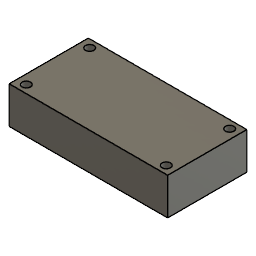
control_dcdc_v0_1 (Autodesk Fusion 360 design; units mm, degrees)
part number: 2026-05-28-15-22-03-641
Autodesk Fusion 360 part; units mm, degrees
box "长方体基本要素1" add length 30 width 60 height 14 placed x (0, 0, 1) y (1, 0, 0) z (0, 1, 0) at (0, 0, 0)
sketch "草图2" plane through (0, 14, 0) normal (0, 1, 0) x (-1, 0, 0)
  line L0 (0, 30) -> (-60, 30)
  line L1 (-60, 30) -> (-60, 0)
  line L2 (-60, 0) -> (0, 0)
  line L3 (0, 0) -> (0, 30)
  circle A0 centre (-3.5, 3) radius 1.6
  circle A1 centre (-3.5, 27) radius 1.6
  circle A2 centre (-56.5, 3) radius 1.6
  circle A3 centre (-56.5, 27) radius 1.6
  line L4 (3.6215, 15) -> (-73.595, 15) construction
  line L5 (-30, -5.3507) -> (-30, 35.2179) construction
  point P0 (0, 15)
  point P1 (-30, 0)
  dimension "d8" = 3.2
  dimension "d9" = 53
  dimension "d10" = 24
  constraint equal A1 A3
  constraint equal A0 A3
  constraint equal A2 A3
  constraint perpendicular L3 L4
  constraint coincident L3 P0
  constraint coincident L2 P1
  constraint midpoint L3 P0
  constraint midpoint L2 P1
  constraint coincident L4 P0
  constraint perpendicular L0 L5
  constraint symmetric A1 A3 L5
  constraint symmetric A2 A3 L4
  constraint symmetric A0 A1 L4
  constraint symmetric A0 A2 L5
  constraint coincident P1 L5
  measures "d8" diameter of A3
  measures "d9" distance of A1.centre A3.centre
  measures "d10" distance of A2.centre A3.centre
extrude "拉伸1" cut sketch "草图2" against normal blind 22 contours A0 | A1 | A2 | A3
